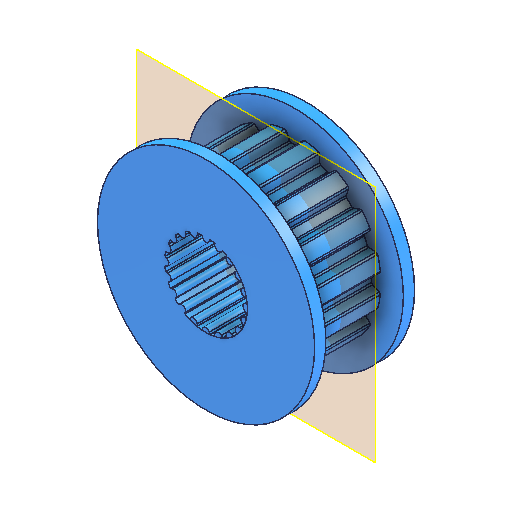
# Autodesk Inventor part: Diff Small Pulley
Saved by Autodesk Inventor 2025.2 (Build 292293000, 293)
## iProperties
Created: 2025-02-20
Part Number: Diff Small Pulley
Material: Generic
Document SubType Name: Modeling
Designer: Jakeg
Density: 1 g/cm^3
Appearance: PTFE
Author: Jakeg
Autodesk Inventor part; units mm, degrees
ref_plane "YZ Plane" through (0, 0, 0) normal (1, 0, 0) x (0, 1, 0)
ref_plane "XZ Plane" through (0, 0, 0) normal (0, 1, 0) x (-1, 0, 0)
ref_plane "XY Plane" through (0, 0, 0) normal (0, 0, 1) x (1, 0, 0)
sketch "Sketch1" plane through (0, 0, 0) normal (0, 0, 1) x (1, 0, 0)
  circle A0 centre (0, 0) radius 6
  circle A1 centre (0, 0) radius 15.75
  dimension "d0" = 12
  dimension "d1" = 31.5
  constraints: 2 centre point, 2 coincident
  measures "d0" diameter of A0
  measures "d1" diameter of A1
extrude "Extrusion1" add sketch "Sketch1" along normal blind 14.5
ref_plane "Work Plane1" through (0, 0, 7.25) normal (0, 0, 1) x (1, 0, 0)
sketch "Sketch2" plane through (0, 0, 7.25) normal (0, 0, 1) x (1, 0, 0)
  circle A0 centre (0, 0) radius 12.5
  circle A1 centre (0, 0) radius 15.75
  dimension "d5" = 25
  constraints: 2 centre point, 2 coincident
  measures "d5" diameter of A0
extrude "Extrusion2" cut sketch "Sketch2" along normal mid plane 11.25
sketch "Sketch3" plane through (0, 0, 14.5) normal (0, 0, 1) x (1, 0, 0)
  arc A0 (-1.278, -5.5468) -> (-2.2269, -5.2385) centre (-1.8276, -5.624) ccw
  arc A1 (-1.2786, -5.8288) -> (-1.278, -5.5468) centre (-2.2683, -5.6858) ccw
  arc A2 (-1.2786, -5.8288) -> (-1.1586, -5.9976) centre (-1.1301, -5.8503) ccw
  arc A3 (-1.1586, -5.9976) -> (-0.7517, -6.062) centre (0, 0) ccw
  arc A4 (-0.7517, -6.062) -> (-0.5855, -5.9386) centre (-0.7333, -5.9131) ccw
  arc A5 (-0.4989, -5.6702) -> (-0.5855, -5.9386) centre (0.4, -6.1084) ccw
  arc A6 (0.4989, -5.6702) -> (-0.4989, -5.6702) centre (0, -5.9134) ccw
  arc A7 (0.5855, -5.9386) -> (0.4989, -5.6702) centre (-0.4, -6.1084) ccw
  arc A8 (0.5855, -5.9386) -> (0.7518, -6.062) centre (0.7333, -5.9131) ccw
  arc A9 (0.7518, -6.062) -> (1.1583, -5.9976) centre (0, 0.0001) ccw
  arc A10 (1.1583, -5.9976) -> (1.2783, -5.8289) centre (1.1299, -5.8503) ccw
  arc A11 (1.2778, -5.5469) -> (1.2783, -5.8289) centre (2.2681, -5.6859) ccw
  arc A12 (2.2267, -5.2385) -> (1.2778, -5.5469) centre (1.8274, -5.624) ccw
  arc A13 (2.392, -5.467) -> (2.2267, -5.2385) centre (1.5072, -5.9331) ccw
  arc A14 (2.392, -5.467) -> (2.5883, -5.533) centre (2.5247, -5.3971) ccw
  arc A15 (2.5883, -5.533) -> (2.955, -5.3461) centre (0, 0.0001) ccw
  arc A16 (2.955, -5.3461) -> (3.017, -5.1486) centre (2.8825, -5.2148) ccw
  arc A17 (2.9293, -4.8805) -> (3.017, -5.1486) centre (3.9141, -4.7067) ccw
  arc A18 (3.7365, -4.2941) -> (2.9293, -4.8805) centre (3.4759, -4.7841) ccw
  arc A19 (3.9643, -4.4603) -> (3.7365, -4.2941) centre (3.2669, -5.1769) ccw
  arc A20 (3.9643, -4.4603) -> (4.1714, -4.4624) centre (4.069, -4.3528) ccw
  arc A21 (4.1714, -4.4624) -> (4.4625, -4.1713) centre (0, 0.0001) ccw
  arc A22 (4.4625, -4.1713) -> (4.4604, -3.9643) centre (4.3529, -4.0689) ccw
  arc A23 (4.2941, -3.7364) -> (4.4604, -3.9643) centre (5.177, -3.2668) ccw
  arc A24 (4.8806, -2.9292) -> (4.2941, -3.7364) centre (4.7841, -3.4758) ccw
  arc A25 (5.1486, -3.0169) -> (4.8806, -2.9292) centre (4.7068, -3.914) ccw
  arc A26 (5.1486, -3.0169) -> (5.3462, -2.9549) centre (5.2149, -2.8824) ccw
  arc A27 (5.3462, -2.9549) -> (5.5331, -2.5882) centre (0, 0.0001) ccw
  arc A28 (5.5331, -2.5882) -> (5.4671, -2.3919) centre (5.3972, -2.5246) ccw
  arc A29 (5.2386, -2.2266) -> (5.4671, -2.3919) centre (5.9331, -1.5071) ccw
  arc A30 (5.5469, -1.2777) -> (5.2386, -2.2266) centre (5.6241, -1.8273) ccw
  arc A31 (5.8289, -1.2783) -> (5.5469, -1.2777) centre (5.6859, -2.268) ccw
  arc A32 (5.8289, -1.2783) -> (5.9977, -1.1582) centre (5.8504, -1.1298) ccw
  arc A33 (5.9977, -1.1582) -> (6.0621, -0.7517) centre (0, 0.0001) ccw
  arc A34 (6.0621, -0.7517) -> (5.9387, -0.5854) centre (5.9132, -0.7332) ccw
  arc A35 (5.6639, -0.4959) -> (5.9387, -0.5854) centre (6.1078, 0.4002) ccw
  arc A36 (5.6639, 0.5019) -> (5.6639, -0.4959) centre (5.9071, 0.003) ccw
  arc A37 (5.9323, 0.5885) -> (5.6639, 0.5019) centre (6.1021, -0.397) ccw
  arc A38 (5.9323, 0.5885) -> (6.0557, 0.7547) centre (5.9068, 0.7363) ccw
  arc A39 (6.0557, 0.7547) -> (5.9913, 1.1613) centre (-0.0064, 0.003) ccw
  arc A40 (5.9913, 1.1613) -> (5.8226, 1.2813) centre (5.844, 1.1329) ccw
  arc A41 (5.5405, 1.2808) -> (5.8226, 1.2813) centre (5.6795, 2.271) ccw
  arc A42 (5.2322, 2.2297) -> (5.5405, 1.2808) centre (5.6177, 1.8304) ccw
  arc A43 (5.4607, 2.395) -> (5.2322, 2.2297) centre (5.9267, 1.5102) ccw
  arc A44 (5.4607, 2.395) -> (5.5267, 2.5912) centre (5.3908, 2.5277) ccw
  arc A45 (5.5267, 2.5912) -> (5.3398, 2.958) centre (-0.0064, 0.003) ccw
  arc A46 (5.3398, 2.958) -> (5.1422, 3.02) centre (5.2085, 2.8854) ccw
  arc A47 (4.8742, 2.9323) -> (5.1422, 3.02) centre (4.7004, 3.9171) ccw
  arc A48 (4.2877, 3.7395) -> (4.8742, 2.9323) centre (4.7777, 3.4789) ccw
  arc A49 (4.454, 3.9673) -> (4.2877, 3.7395) centre (5.1706, 3.2699) ccw
  arc A50 (4.454, 3.9673) -> (4.4561, 4.1744) centre (4.3465, 4.0719) ccw
  arc A51 (4.4561, 4.1744) -> (4.165, 4.4654) centre (-0.0064, 0.003) ccw
  arc A52 (4.165, 4.4654) -> (3.9579, 4.4634) centre (4.0626, 4.3559) ccw
  arc A53 (3.7301, 4.2971) -> (3.9579, 4.4634) centre (3.2605, 5.18) ccw
  arc A54 (2.9229, 4.8836) -> (3.7301, 4.2971) centre (3.4695, 4.7871) ccw
  arc A55 (3.0106, 5.1516) -> (2.9229, 4.8836) centre (3.9077, 4.7098) ccw
  arc A56 (3.0106, 5.1516) -> (2.9486, 5.3492) centre (2.8761, 5.2179) ccw
  arc A57 (2.9486, 5.3492) -> (2.5819, 5.5361) centre (-0.0064, 0.003) ccw
  arc A58 (2.5819, 5.5361) -> (2.3856, 5.4701) centre (2.5183, 5.4002) ccw
  arc A59 (2.2203, 5.2416) -> (2.3856, 5.4701) centre (1.5008, 5.9361) ccw
  arc A60 (1.2714, 5.5499) -> (2.2203, 5.2416) centre (1.821, 5.6271) ccw
  arc A61 (1.2719, 5.8319) -> (1.2714, 5.5499) centre (2.2617, 5.6889) ccw
  arc A62 (1.2719, 5.8319) -> (1.1519, 6.0007) centre (1.1235, 5.8534) ccw
  arc A63 (1.1519, 6.0007) -> (0.7454, 6.0651) centre (-0.0064, 0.003) ccw
  arc A64 (0.7454, 6.0651) -> (0.5791, 5.9417) centre (0.7269, 5.9162) ccw
  arc A65 (0.4925, 5.6733) -> (0.5791, 5.9417) centre (-0.4064, 6.1115) ccw
  arc A66 (-0.5053, 5.6733) -> (0.4925, 5.6733) centre (-0.0064, 5.9165) ccw
  arc A67 (-0.5919, 5.9417) -> (-0.5053, 5.6733) centre (0.3936, 6.1115) ccw
  arc A68 (-0.5919, 5.9417) -> (-0.7581, 6.0651) centre (-0.7397, 5.9162) ccw
  arc A69 (-0.7581, 6.0651) -> (-1.1647, 6.0007) centre (-0.0064, 0.003) ccw
  arc A70 (-1.1647, 6.0007) -> (-1.2847, 5.8319) centre (-1.1363, 5.8534) ccw
  arc A71 (-1.2841, 5.5499) -> (-1.2847, 5.8319) centre (-2.2744, 5.6889) ccw
  arc A72 (-2.2331, 5.2416) -> (-1.2841, 5.5499) centre (-1.8338, 5.6271) ccw
  arc A73 (-2.3984, 5.4701) -> (-2.2331, 5.2416) centre (-1.5136, 5.9361) ccw
  arc A74 (-2.3984, 5.4701) -> (-2.5946, 5.5361) centre (-2.5311, 5.4002) ccw
  arc A75 (-2.5946, 5.5361) -> (-2.9614, 5.3492) centre (-0.0064, 0.003) ccw
  arc A76 (-2.9614, 5.3492) -> (-3.0234, 5.1516) centre (-2.8888, 5.2179) ccw
  arc A77 (-2.9357, 4.8836) -> (-3.0234, 5.1516) centre (-3.9205, 4.7098) ccw
  arc A78 (-3.7429, 4.2971) -> (-2.9357, 4.8836) centre (-3.4823, 4.7871) ccw
  arc A79 (-3.9707, 4.4634) -> (-3.7429, 4.2971) centre (-3.2733, 5.18) ccw
  arc A80 (-3.9707, 4.4634) -> (-4.1778, 4.4654) centre (-4.0753, 4.3559) ccw
  arc A81 (-4.1778, 4.4654) -> (-4.4688, 4.1744) centre (-0.0064, 0.003) ccw
  arc A82 (-4.4688, 4.1744) -> (-4.4667, 3.9673) centre (-4.3592, 4.0719) ccw
  arc A83 (-4.3005, 3.7395) -> (-4.4667, 3.9673) centre (-5.1834, 3.2699) ccw
  arc A84 (-4.887, 2.9323) -> (-4.3005, 3.7395) centre (-4.7905, 3.4789) ccw
  arc A85 (-5.155, 3.02) -> (-4.887, 2.9323) centre (-4.7132, 3.9171) ccw
  arc A86 (-5.155, 3.02) -> (-5.3526, 2.958) centre (-5.2213, 2.8854) ccw
  arc A87 (-5.3526, 2.958) -> (-5.5394, 2.5912) centre (-0.0064, 0.003) ccw
  arc A88 (-5.5394, 2.5912) -> (-5.4735, 2.395) centre (-5.4036, 2.5277) ccw
  arc A89 (-5.245, 2.2297) -> (-5.4735, 2.395) centre (-5.9395, 1.5102) ccw
  arc A90 (-5.5533, 1.2808) -> (-5.245, 2.2297) centre (-5.6305, 1.8304) ccw
  arc A91 (-5.8353, 1.2813) -> (-5.5533, 1.2808) centre (-5.6923, 2.271) ccw
  arc A92 (-5.8353, 1.2813) -> (-6.0041, 1.1613) centre (-5.8568, 1.1329) ccw
  arc A93 (-6.0041, 1.1613) -> (-6.0685, 0.7547) centre (-0.0064, 0.003) ccw
  arc A94 (-6.0685, 0.7547) -> (-5.9451, 0.5885) centre (-5.9196, 0.7363) ccw
  arc A95 (-5.6767, 0.5019) -> (-5.9451, 0.5885) centre (-6.1149, -0.397) ccw
  arc A96 (-5.6767, -0.4959) -> (-5.6767, 0.5019) centre (-5.9199, 0.003) ccw
  arc A97 (-5.9451, -0.5825) -> (-5.6767, -0.4959) centre (-6.1149, 0.403) ccw
  arc A98 (-5.9451, -0.5825) -> (-6.0685, -0.7488) centre (-5.9196, -0.7303) ccw
  arc A99 (-6.0685, -0.7488) -> (-6.0041, -1.1553) centre (-0.0064, 0.003) ccw
  arc A100 (-6.0041, -1.1553) -> (-5.8353, -1.2753) centre (-5.8568, -1.1269) ccw
  arc A101 (-5.5533, -1.2748) -> (-5.8353, -1.2753) centre (-5.6923, -2.2651) ccw
  arc A102 (-5.245, -2.2237) -> (-5.5533, -1.2748) centre (-5.6305, -1.8244) ccw
  arc A103 (-5.4735, -2.389) -> (-5.245, -2.2237) centre (-5.9395, -1.5042) ccw
  arc A104 (-5.4735, -2.389) -> (-5.5394, -2.5853) centre (-5.4036, -2.5217) ccw
  arc A105 (-5.5394, -2.5853) -> (-5.3526, -2.952) centre (-0.0064, 0.003) ccw
  arc A106 (-5.3526, -2.952) -> (-5.155, -3.014) centre (-5.2213, -2.8795) ccw
  arc A107 (-4.887, -2.9263) -> (-5.155, -3.014) centre (-4.7132, -3.9111) ccw
  arc A108 (-4.3005, -3.7335) -> (-4.887, -2.9263) centre (-4.7905, -3.4729) ccw
  arc A109 (-4.4667, -3.9613) -> (-4.3005, -3.7335) centre (-5.1834, -3.2639) ccw
  arc A110 (-4.4667, -3.9613) -> (-4.4688, -4.1684) centre (-4.3592, -4.066) ccw
  arc A111 (-4.4688, -4.1684) -> (-4.1778, -4.4594) centre (-0.0064, 0.003) ccw
  arc A112 (-4.1778, -4.4594) -> (-3.9707, -4.4574) centre (-4.0753, -4.3499) ccw
  arc A113 (-3.7429, -4.2911) -> (-3.9707, -4.4574) centre (-3.2733, -5.174) ccw
  arc A114 (-2.9357, -4.8776) -> (-3.7429, -4.2911) centre (-3.4823, -4.7811) ccw
  arc A115 (-3.0234, -5.1456) -> (-2.9357, -4.8776) centre (-3.9205, -4.7038) ccw
  arc A116 (-3.0234, -5.1456) -> (-2.9614, -5.3432) centre (-2.8888, -5.2119) ccw
  arc A117 (-2.9614, -5.3432) -> (-2.5885, -5.5329) centre (-0.006, 0.0037) ccw
  arc A118 (-2.5885, -5.5329) -> (-2.3922, -5.467) centre (-2.5249, -5.3971) ccw
  arc A119 (-2.2269, -5.2385) -> (-2.3922, -5.467) centre (-1.5074, -5.933) ccw
  circle A120 centre (-0.006, 0.0037) radius 6
  circle A121 centre (-0.006, 0.0037) radius 12.5204
  arc A122 (-9.7164, 7.9073) -> (-9.7028, 7.7034) centre (-9.6001, 7.8127) ccw
  arc A123 (-9.5366, 7.4755) -> (-9.7028, 7.7034) centre (-10.4195, 7.0059) ccw
  arc A124 (-10.1231, 6.6683) -> (-9.5366, 7.4755) centre (-10.0266, 7.2149) ccw
  arc A125 (-10.3911, 6.756) -> (-10.1231, 6.6683) centre (-9.9492, 7.6531) ccw
  arc A126 (-10.3911, 6.756) -> (-10.5841, 6.7017) centre (-10.4574, 6.6215) ccw
  arc A127 (-11.383, 4.9039) -> (-11.5641, 4.8177) centre (-11.4256, 4.76) ccw
  arc A128 (-11.383, 4.9039) -> (-11.104, 4.8627) centre (-11.0991, 5.8627) ccw
  arc A129 (-11.104, 4.8627) -> (-10.6624, 5.7574) centre (-11.1013, 5.4177) ccw
  arc A130 (-10.9126, 6.1526) -> (-10.8647, 5.9539) centre (-10.7819, 6.079) ccw
  arc A131 (-10.6624, 5.7574) -> (-10.8647, 5.9539) centre (-11.4532, 5.1454) ccw
  arc A132 (-12.0476, 2.9107) -> (-12.2115, 2.7952) centre (-12.0653, 2.7618) ccw
  arc A133 (-12.0476, 2.9107) -> (-11.7657, 2.9173) centre (-11.9298, 3.9038) ccw
  arc A134 (-11.7657, 2.9173) -> (-11.4816, 3.8738) centre (-11.8568, 3.4648) ccw
  arc A135 (-11.795, 4.221) -> (-11.7143, 4.0332) centre (-11.6538, 4.1705) ccw
  arc A136 (-11.4816, 3.8738) -> (-11.7143, 4.0332) centre (-12.1576, 3.1369) ccw
  arc A137 (-12.3658, 0.8339) -> (-12.5078, 0.6924) centre (-12.3581, 0.6841) ccw
  arc A138 (-12.3658, 0.8339) -> (-12.0891, 0.8881) centre (-12.4176, 1.8326) ccw
  arc A139 (-12.0891, 0.8881) -> (-11.9707, 1.8788) centre (-12.2714, 1.4123) ccw
  arc A140 (-12.3383, 2.1681) -> (-12.227, 1.9966) centre (-12.1906, 2.1421) ccw
  arc A141 (-11.9707, 1.8788) -> (-12.227, 1.9966) centre (-12.5124, 1.0382) ccw
  arc A142 (-12.3285, -1.2668) -> (-12.4445, -1.4303) centre (-12.2955, -1.4131) ccw
  arc A143 (-12.3285, -1.2668) -> (-12.0648, -1.1666) centre (-12.5483, -0.2912) ccw
  arc A144 (-12.0648, -1.1666) -> (-12.1157, -0.1702) centre (-12.3331, -0.6808) ccw
  arc A145 (-12.5268, 0.0528) -> (-12.3881, -0.0974) centre (-12.3768, 0.0522) ccw
  arc A146 (-12.1157, -0.1702) -> (-12.3881, -0.0974) centre (-12.5075, -1.0902) ccw
  arc A147 (-11.9366, -3.331) -> (-12.0234, -3.5117) centre (-11.8794, -3.4696) ccw
  arc A148 (-11.9366, -3.331) -> (-11.6937, -3.1877) centre (-12.3181, -2.4066) ccw
  arc A149 (-11.6937, -3.1877) -> (-11.9122, -2.2142) centre (-12.0403, -2.7542) ccw
  arc A150 (-12.3551, -2.0639) -> (-12.193, -2.1884) centre (-12.2072, -2.0391) ccw
  arc A151 (-11.9122, -2.2142) -> (-12.193, -2.1884) centre (-12.1429, -3.1872) ccw
  arc A152 (-11.2016, -5.2992) -> (-11.2565, -5.4921) centre (-11.1218, -5.4262) ccw
  arc A153 (-11.2016, -5.2992) -> (-10.9864, -5.117) centre (-11.7338, -4.4526) ccw
  arc A154 (-10.9864, -5.117) -> (-11.3663, -4.1944) centre (-11.4012, -4.7483) ccw
  arc A155 (-11.8282, -4.1211) -> (-11.6474, -4.2165) centre (-11.6866, -4.0717) ccw
  arc A156 (-11.3663, -4.1944) -> (-11.6474, -4.2165) centre (-11.4292, -5.1924) ccw
  arc A157 (-10.1445, -7.115) -> (-10.166, -7.3143) centre (-10.0443, -7.2266) ccw
  arc A158 (-10.1445, -7.115) -> (-9.9632, -6.899) centre (-10.8121, -6.3705) ccw
  arc A159 (-9.9632, -6.899) -> (-10.4935, -6.0538) centre (-10.4343, -6.6057) ccw
  arc A160 (-10.9612, -6.0597) -> (-10.7669, -6.1231) centre (-10.83, -5.987) ccw
  arc A161 (-10.4935, -6.0538) -> (-10.7669, -6.1231) centre (-10.3869, -7.0481) ccw
  arc A162 (-8.7957, -8.7259) -> (-8.7833, -8.926) centre (-8.6781, -8.8191) ccw
  arc A163 (-8.7957, -8.7259) -> (-8.6535, -8.4824) centre (-9.5796, -8.105) ccw
  arc A164 (-8.6535, -8.4824) -> (-9.319, -7.739) centre (-9.1675, -8.2729) ccw
  arc A165 (-9.779, -7.8238) -> (-9.5768, -7.8535) centre (-9.662, -7.7301) ccw
  arc A166 (-9.319, -7.739) -> (-9.5768, -7.8535) centre (-9.0459, -8.701) ccw
  arc A167 (-7.1941, -10.0858) -> (-7.148, -10.2809) centre (-7.0625, -10.1577) ccw
  arc A168 (-7.1941, -10.0858) -> (-7.0951, -9.8217) centre (-8.0716, -9.6062) ccw
  arc A169 (-7.0951, -9.8217) -> (-7.8767, -9.2015) centre (-7.6371, -9.7021) ccw
  arc A170 (-8.3157, -9.3628) -> (-8.1113, -9.3579) centre (-8.2162, -9.2506) ccw
  arc A171 (-7.8767, -9.2015) -> (-8.1113, -9.3579) centre (-7.4449, -10.1035) ccw
  arc A172 (-5.3857, -11.1554) -> (-5.3073, -11.3399) centre (-5.2438, -11.204) ccw
  arc A173 (-5.3857, -11.1554) -> (-5.3328, -10.8784) centre (-6.3316, -10.831) ccw
  arc A174 (-5.3328, -10.8784) -> (-6.2079, -10.3992) centre (-5.8871, -10.8521) ccw
  arc A175 (-6.6134, -10.6324) -> (-6.4128, -10.593) centre (-6.5342, -10.505) ccw
  arc A176 (-6.2079, -10.3992) -> (-6.4128, -10.593) centre (-5.6299, -11.2153) ccw
  arc A177 (-3.4225, -11.904) -> (-3.3141, -12.0726) centre (-3.2745, -11.9279) ccw
  arc A178 (-3.4225, -11.904) -> (-3.4172, -11.622) centre (-4.4097, -11.7442) ccw
  arc A179 (-3.4172, -11.622) -> (-4.3607, -11.2976) centre (-3.968, -11.6898) ccw
  arc A180 (-4.7209, -11.596) -> (-4.5299, -11.5233) centre (-4.6645, -11.457) ccw
  arc A181 (-4.3607, -11.2976) -> (-4.5299, -11.5233) centre (-3.6531, -12.0043) ccw
  arc A182 (-1.3611, -12.31) -> (-1.2257, -12.4579) centre (-1.2111, -12.3086) ccw
  arc A183 (-1.3611, -12.31) -> (-1.4035, -12.0312) centre (-2.3611, -12.3194) ccw
  arc A184 (-1.4035, -12.0312) -> (-2.3883, -11.871) centre (-1.9349, -12.1911) ccw
  arc A185 (-2.6929, -12.2259) -> (-2.5169, -12.122) centre (-2.6607, -12.0794) ccw
  arc A186 (-2.3883, -11.871) -> (-2.5169, -12.122) centre (-1.5715, -12.4479) ccw
  arc A187 (0.7393, -12.3619) -> (0.8977, -12.4848) centre (0.8869, -12.3352) ccw
  arc A188 (0.7393, -12.3619) -> (0.6504, -12.0942) centre (-0.2447, -12.5401) ccw
  arc A189 (0.6504, -12.0942) -> (-0.3473, -12.1027) centre (0.1536, -12.3417) ccw
  arc A190 (-0.5875, -12.5041) -> (-0.4316, -12.3718) centre (-0.5806, -12.3542) ccw
  arc A191 (-0.3473, -12.1027) -> (-0.4316, -12.3718) centre (0.5553, -12.5333) ccw
  arc A192 (2.8182, -12.058) -> (2.9952, -12.1523) centre (2.9592, -12.0067) ccw
  arc A193 (2.8182, -12.058) -> (2.6854, -11.8092) centre (1.8785, -12.3999) ccw
  arc A194 (2.6854, -11.8092) -> (1.7035, -11.9862) centre (2.2376, -12.1371) ccw
  arc A195 (1.5345, -12.4224) -> (1.6658, -12.2657) centre (1.5161, -12.2735) ccw
  arc A196 (1.7035, -11.9862) -> (1.6658, -12.2657) centre (2.6658, -12.258) ccw
  arc A197 (4.8159, -11.4072) -> (5.0062, -11.4702) centre (4.9462, -11.3328) ccw
  arc A198 (4.8159, -11.4072) -> (4.643, -11.1844) centre (3.9475, -11.903) ccw
  arc A199 (4.643, -11.1844) -> (3.7051, -11.5248) centre (4.257, -11.5832) ccw
  arc A200 (3.6123, -11.9832) -> (3.7152, -11.8066) centre (3.5689, -11.8396) ccw
  arc A201 (3.7051, -11.5248) -> (3.7152, -11.8066) centre (4.6995, -11.6301) ccw
  arc A202 (6.6749, -10.4281) -> (6.8731, -10.4581) centre (6.7907, -10.3327) ccw
  arc A203 (6.6749, -10.4281) -> (6.4668, -10.2377) centre (5.9027, -11.0635) ccw
  arc A204 (6.4668, -10.2377) -> (5.5999, -10.7317) centre (6.1537, -10.696) ccw
  arc A205 (5.5859, -11.1993) -> (5.6575, -11.0078) centre (5.5189, -11.0651) ccw
  arc A206 (5.5999, -10.7317) -> (5.6575, -11.0078) centre (6.5978, -10.6674) ccw
  arc A207 (8.3416, -9.1489) -> (8.5421, -9.1449) centre (8.4397, -9.0354) ccw
  arc A208 (8.3416, -9.1489) -> (8.1044, -8.9965) centre (7.688, -9.9057) ccw
  arc A209 (8.1044, -8.9965) -> (7.3334, -9.6299) centre (7.8733, -9.5011) ccw
  arc A210 (7.3986, -10.093) -> (7.4369, -9.8922) centre (7.3099, -9.9721) ccw
  arc A211 (7.3334, -9.6299) -> (7.4369, -9.8922) centre (8.3061, -9.3978) ccw
  arc A212 (9.7682, -7.6064) -> (9.9651, -7.5687) centre (9.8457, -7.478) ccw
  arc A213 (9.7682, -7.6064) -> (9.5086, -7.4963) centre (9.2519, -8.4628) ccw
  arc A214 (9.5086, -7.4963) -> (8.8558, -8.2509) centre (9.3661, -8.0327) ccw
  arc A215 (8.9984, -8.6963) -> (9.0021, -8.4919) centre (8.8905, -8.5921) ccw
  arc A216 (8.8558, -8.2509) -> (9.0021, -8.4919) centre (9.7753, -7.8578) ccw
  arc A217 (10.9136, -5.845) -> (11.1013, -5.7745) centre (10.9683, -5.7053) ccw
  arc A218 (10.9136, -5.845) -> (10.6391, -5.7804) centre (10.5494, -6.7764) ccw
  arc A219 (10.6391, -5.7804) -> (10.1232, -6.6344) centre (10.5893, -6.3332) ccw
  arc A220 (10.339, -7.0494) -> (10.3082, -6.8473) centre (10.2151, -6.9649) ccw
  arc A221 (10.1232, -6.6344) -> (10.3082, -6.8473) centre (10.9631, -6.0916) ccw
  arc A222 (11.7449, -3.9154) -> (11.918, -3.8142) centre (11.7751, -3.7685) ccw
  arc A223 (11.7449, -3.9154) -> (11.4634, -3.8981) centre (11.5433, -4.8949) ccw
  arc A224 (11.4634, -3.8981) -> (11.0993, -4.827) centre (11.5078, -4.4513) ccw
  arc A225 (11.3821, -5.1996) -> (11.3175, -5.0056) centre (11.2456, -5.1373) ccw
  arc A226 (11.0993, -4.827) -> (11.3175, -5.0056) centre (11.8353, -4.1501) ccw
  arc A227 (12.2381, -1.8731) -> (12.3916, -1.7441) centre (12.243, -1.7232) ccw
  arc A228 (12.2381, -1.8731) -> (11.9577, -1.9036) centre (12.2049, -2.8725) ccw
  arc A229 (11.9577, -1.9036) -> (11.7558, -2.8807) centre (12.0949, -2.4414) ccw
  arc A230 (12.0975, -3.2001) -> (12.0011, -3.0198) centre (11.9525, -3.1617) ccw
  arc A231 (11.7558, -2.8807) -> (12.0011, -3.0198) centre (12.3668, -2.0891) ccw
  arc A232 (12.379, 0.2232) -> (12.5085, 0.3763) centre (12.3586, 0.3718) ccw
  arc A233 (12.379, 0.2232) -> (12.1078, 0.1458) centre (12.5153, -0.7675) ccw
  arc A234 (12.1078, 0.1458) -> (12.0739, -0.8514) centre (12.3339, -0.3611) ccw
  arc A235 (12.4647, -1.1084) -> (12.3392, -0.9471) centre (12.3153, -1.0951) ccw
  arc A236 (12.0739, -0.8514) -> (12.3392, -0.9471) centre (12.5424, 0.0321) ccw
  arc A237 (12.1636, 2.3132) -> (12.2654, 2.486) centre (12.1184, 2.4562) ccw
  arc A238 (12.1636, 2.3132) -> (11.9094, 2.191) centre (12.4653, 1.3598) ccw
  arc A239 (11.9094, 2.191) -> (12.0446, 1.2025) centre (12.218, 1.7297) ccw
  arc A240 (12.4732, 1.0152) -> (12.3222, 1.153) centre (12.3237, 1.003) ccw
  arc A241 (12.0446, 1.2025) -> (12.3222, 1.153) centre (12.357, 2.1524) ccw
  arc A242 (11.5981, 4.3367) -> (11.6692, 4.5242) centre (11.5294, 4.47) ccw
  arc A243 (11.5981, 4.3367) -> (11.3683, 4.1733) centre (12.0567, 3.448) ccw
  arc A244 (11.3683, 4.1733) -> (11.6685, 3.2218) centre (11.7503, 3.7708) ccw
  arc A245 (12.1226, 3.1097) -> (11.9505, 3.22) centre (11.9773, 3.0724) ccw
  arc A246 (11.6685, 3.2218) -> (11.9505, 3.22) centre (11.8159, 4.2109) ccw
  arc A247 (10.6988, 6.2355) -> (10.7372, 6.4323) centre (10.6085, 6.3553) ccw
  arc A248 (10.6988, 6.2355) -> (10.4999, 6.0357) centre (11.3009, 5.4371) ccw
  arc A249 (10.4999, 6.0357) -> (10.9566, 5.1486) centre (10.9444, 5.7035) ccw
  arc A250 (11.4231, 5.1148) -> (11.2348, 5.1945) centre (11.2862, 5.0535) ccw
  arc A251 (10.9566, 5.1486) -> (11.2348, 5.1945) centre (10.9347, 6.1484) ccw
  arc A252 (9.4915, 7.9551) -> (9.4961, 8.1555) centre (9.3823, 8.0579) ccw
  arc A253 (9.4915, 7.9551) -> (9.3292, 7.7245) centre (10.2199, 7.2699) ccw
  arc A254 (9.3292, 7.7245) -> (9.9293, 6.9274) centre (9.8235, 7.4722) ccw
  arc A255 (10.3948, 6.9729) -> (10.1958, 7.0196) centre (10.2702, 6.8893) ccw
  arc A256 (9.9293, 6.9274) -> (10.1958, 7.0196) centre (9.7388, 7.909) ccw
  arc A257 (8.011, 9.4458) -> (7.9816, 9.6442) centre (7.886, 9.5287) ccw
  arc A258 (8.011, 9.4458) -> (7.89, 9.1911) centre (8.8447, 8.8936) ccw
  arc A259 (7.89, 9.1911) -> (8.6162, 8.5069) centre (8.4199, 9.026) ccw
  arc A260 (9.0673, 8.6304) -> (8.8632, 8.6428) centre (8.9586, 8.527) ccw
  arc A261 (8.6162, 8.5069) -> (8.8632, 8.6428) centre (8.2625, 9.4422) ccw
  arc A262 (6.2998, 10.665) -> (6.2374, 10.8555) centre (6.1626, 10.7255) ccw
  arc A263 (6.2998, 10.665) -> (6.2236, 10.3935) centre (7.2149, 10.2616) ccw
  arc A264 (6.2236, 10.3935) -> (7.055, 9.8418) centre (6.7737, 10.3203) ccw
  arc A265 (7.4787, 10.0398) -> (7.2755, 10.0175) centre (7.3891, 9.9195) ccw
  arc A266 (7.055, 9.8418) -> (7.2755, 10.0175) centre (6.5483, 10.7039) ccw
  arc A267 (4.4072, 11.5774) -> (4.3135, 11.7546) centre (4.2617, 11.6138) ccw
  arc A268 (4.4072, 11.5774) -> (4.378, 11.2969) centre (5.3773, 11.3344) ccw
  arc A269 (4.378, 11.2969) -> (5.2906, 10.8936) centre (4.9326, 11.3177) ccw
  arc A270 (5.6748, 11.1604) -> (5.4783, 11.1041) centre (5.6068, 11.0267) ccw
  arc A271 (5.2906, 10.8936) -> (5.4783, 11.1041) centre (4.6455, 11.6577) ccw
  arc A272 (2.3877, 12.1568) -> (2.2653, 12.3156) centre (2.2381, 12.1681) ccw
  arc A273 (2.3877, 12.1568) -> (2.4062, 11.8754) centre (3.3848, 12.0813) ccw
  arc A274 (2.4062, 11.8754) -> (3.3739, 11.6322) centre (2.9494, 11.9896) ccw
  arc A275 (3.7075, 11.96) -> (3.5233, 11.8714) centre (3.663, 11.8168) ccw
  arc A276 (3.3739, 11.6322) -> (3.5233, 11.8714) centre (2.609, 12.2763) ccw
  arc A277 (0.2992, 12.3866) -> (0.1518, 12.5224) centre (0.1499, 12.3724) ccw
  arc A278 (0.2992, 12.3866) -> (0.3651, 12.1123) centre (1.2948, 12.4806) ccw
  arc A279 (0.3651, 12.1123) -> (1.3599, 12.0362) centre (0.8811, 12.3168) ccw
  arc A280 (1.6333, 12.4157) -> (1.4668, 12.2972) centre (1.6137, 12.267) ccw
  arc A281 (1.3599, 12.0362) -> (1.4668, 12.2972) centre (0.4971, 12.5417) ccw
  arc A282 (-1.798, 12.2601) -> (-1.9663, 12.3691) centre (-1.9428, 12.2209) ccw
  arc A283 (-1.798, 12.2601) -> (-1.6867, 12.0009) centre (-0.8326, 12.5211) ccw
  arc A284 (-1.6867, 12.0009) -> (-0.6933, 12.094) centre (-1.2127, 12.2896) ccw
  arc A285 (-0.488, 12.5143) -> (-0.6321, 12.3693) centre (-0.4822, 12.3644) ccw
  arc A286 (-0.6933, 12.094) -> (-0.6321, 12.3693) centre (-1.6292, 12.4465) ccw
  arc A287 (-3.8437, 11.781) -> (-4.028, 11.86) centre (-3.9798, 11.7179) ccw
  arc A288 (-3.8437, 11.781) -> (-3.6902, 11.5444) centre (-2.9363, 12.2014) ccw
  arc A289 (-3.6902, 11.5444) -> (-2.7268, 11.804) centre (-3.2718, 11.909) ccw
  arc A290 (-2.5955, 12.2529) -> (-2.7131, 12.0857) centre (-2.5645, 12.1062) ccw
  arc A291 (-2.7268, 11.804) -> (-2.7131, 12.0857) centre (-3.7088, 11.9932) ccw
  arc A292 (-5.779, 10.9631) -> (-5.974, 11.0098) centre (-5.9025, 10.8779) ccw
  arc A293 (-5.779, 10.9631) -> (-5.5877, 10.7558) centre (-4.9557, 11.5307) ccw
  arc A294 (-5.5877, 10.7558) -> (-4.6821, 11.1745) centre (-5.237, 11.1859) ccw
  arc A295 (-4.6285, 11.6391) -> (-4.7161, 11.4544) centre (-4.5731, 11.4997) ccw
  arc A296 (-4.6821, 11.1745) -> (-4.7161, 11.4544) centre (-5.6819, 11.195) ccw
  arc A297 (-7.5482, 9.8299) -> (-7.7483, 9.8429) centre (-7.6555, 9.7251) ccw
  arc A298 (-7.5482, 9.8299) -> (-7.3247, 9.6579) centre (-6.8327, 10.5285) ccw
  arc A299 (-7.3247, 9.6579) -> (-6.5028, 10.2236) centre (-7.0517, 10.1411) ccw
  arc A300 (-6.5285, 10.6906) -> (-6.5837, 10.4938) centre (-6.4504, 10.5626) ccw
  arc A301 (-6.5028, 10.2236) -> (-6.5837, 10.4938) centre (-7.4917, 10.0749) ccw
  arc A302 (-9.1005, 8.4139) -> (-9.2999, 8.393) centre (-9.1885, 8.2925) ccw
  arc A303 (-9.1005, 8.4139) -> (-8.8511, 8.2822) centre (-8.5134, 9.2234) ccw
  arc A304 (-8.8511, 8.2822) -> (-8.1367, 8.9787) centre (-8.6637, 8.8046) ccw
  arc A305 (-8.2409, 9.4347) -> (-8.262, 9.2313) centre (-8.1423, 9.3217) ccw
  arc A306 (-8.1367, 8.9787) -> (-8.262, 9.2313) centre (-9.0862, 8.665) ccw
  point P0 (-3.9961, -4.4772)
  point P1 (-3.0344, -5.1759)
  point P2 (-5.1854, -3.0251)
  point P3 (-4.4866, -3.9867)
  point P4 (-5.8678, -1.2765)
  point P5 (-5.5003, -2.4071)
  point P6 (-5.9765, 0.5975)
  point P7 (-5.9764, -0.5915)
  point P8 (-5.5008, 2.4135)
  point P9 (-5.8681, 1.2824)
  point P10 (-4.4872, 3.9936)
  point P11 (-5.1861, 3.0313)
  point P12 (-3.0348, 5.1832)
  point P13 (-3.9971, 4.4838)
  point P14 (-1.2858, 5.8657)
  point P15 (-2.4173, 5.4979)
  point P16 (0.5886, 5.9742)
  point P17 (-0.6013, 5.9741)
  point P18 (2.4047, 5.4982)
  point P19 (1.273, 5.8659)
  point P20 (3.9848, 4.4841)
  point P21 (3.0221, 5.1836)
  point P22 (5.1741, 3.0314)
  point P23 (4.4747, 3.9941)
  point P24 (5.8562, 1.2824)
  point P25 (5.4886, 2.414)
  point P26 (5.9644, -0.5922)
  point P27 (5.9645, 0.5978)
  point P28 (5.4889, -2.4059)
  point P29 (5.8551, -1.2797)
  point P30 (4.4768, -3.9843)
  point P31 (5.1727, -3.0263)
  point P32 (3.0266, -5.1734)
  point P33 (3.9846, -4.4768)
  point P34 (1.2797, -5.8569)
  point P35 (2.4067, -5.4898)
  point P36 (-0.5935, -5.9674)
  point P37 (0.593, -5.9663)
  point P38 (-2.4101, -5.4936)
  point P39 (-1.2798, -5.8595)
  dimension "d8" = 0
  dimension "d9" = 0
  dimension "d20" = 360
  constraints: 612 point on circle, 306 centre point, 3 coincident, 2 tangent, 595 other
  measures "d8" distance of point (0, 0) point (0, 0)
  measures "d9" distance of point (0, 0) point (0, 0)
extrude "Extrusion3" add sketch "Sketch3" against normal blind 14.5 contours A1 A2 A120 A118 A119 A0 | A120 A4 A3 A2 | A118 A117 A116 A120 | A4 A5 A6 A7 A8 A120 | A120 A112 A113 A114 A115 A116 | A120 A10 A9 A8 | A112 A111 A110 A120 | A10 A11 A12 A13 A14 A120 | A120 A106 A107 A108 A109 A110 | A120 A16 A15 A14 | A106 A105 A104 A120 | A16 A17 A18 A19 A20 A120 | A120 A100 A101 A102 A103 A104 | A120 A22 A21 A20 | A100 A99 A98 A120 | A22 A23 A24 A25 A26 A120 | A120 A94 A95 A96 A97 A98 | A120 A28 A27 A26 | A94 A93 A92 A120 | A28 A29 A30 A31 A32 A120 | A120 A88 A89 A90 A91 A92 | A120 A34 A33 A32 | A88 A87 A86 A120 | A34 A35 A36 A37 A38 A120 | A120 A82 A83 A84 A85 A86 | A82 A81 A80 A120 | A120 A40 A39 A38 | A120 A76 A77 A78 A79 A80 | A40 A41 A42 A43 A44 A120 | A76 A75 A74 A120 | A120 A46 A45 A44 | A120 A70 A71 A72 A73 A74 | A46 A47 A48 A49 A50 A120 | A70 A69 A68 A120 | A120 A52 A51 A50 | A120 A64 A65 A66 A67 A68 | A52 A53 A54 A55 A56 A120 | A64 A63 A62 A120 | A120 A58 A57 A56 | A120 A58 A59 A60 A61 A62
sketch "Sketch6" plane through (0, 0, 1.625) normal (0, 0, 1) x (1, 0, 0)
  circle A0 centre (0, 0) radius 14.7498
  line L0 (3.5809, 11.7957) -> (3.627, 10.7394)
  arc A1 (3.627, 10.7394) -> (3.7836, 10.5159) centre (3.8808, 10.7505) ccw
  line L1 (3.7836, 10.5159) -> (4.7604, 10.1112)
  arc A2 (4.7604, 10.1112) -> (5.0292, 10.1586) centre (4.8576, 10.3459) ccw
  line L2 (5.0292, 10.1586) -> (5.8087, 10.8729)
  arc A3 (6.1044, 10.9073) -> (5.8087, 10.8729) centre (5.9803, 10.6856) ccw
  arc A4 (7.741, 9.8138) -> (6.1044, 10.9073) centre (0, 0) ccw
  arc A5 (7.8223, 9.5275) -> (7.741, 9.8138) centre (7.5837, 9.6143) ccw
  line L3 (7.8223, 9.5275) -> (7.4607, 8.534)
  arc A6 (7.4607, 8.534) -> (7.5198, 8.2675) centre (7.6994, 8.4471) ccw
  line L4 (7.5198, 8.2675) -> (8.2675, 7.5198)
  arc A7 (8.2675, 7.5198) -> (8.534, 7.4607) centre (8.4471, 7.6994) ccw
  line L5 (8.534, 7.4607) -> (9.5275, 7.8223)
  arc A8 (9.8138, 7.741) -> (9.5275, 7.8223) centre (9.6143, 7.5837) ccw
  arc A9 (10.9073, 6.1044) -> (9.8138, 7.741) centre (0, 0) ccw
  arc A10 (10.8729, 5.8087) -> (10.9073, 6.1044) centre (10.6856, 5.9803) ccw
  line L6 (10.8729, 5.8087) -> (10.1586, 5.0292)
  arc A11 (10.1586, 5.0292) -> (10.1112, 4.7604) centre (10.3459, 4.8576) ccw
  line L7 (10.1112, 4.7604) -> (10.5159, 3.7836)
  arc A12 (10.5159, 3.7836) -> (10.7394, 3.627) centre (10.7505, 3.8808) ccw
  line L8 (10.7394, 3.627) -> (11.7957, 3.5809)
  arc A13 (12.0291, 3.3962) -> (11.7957, 3.5809) centre (11.7846, 3.3271) ccw
  arc A14 (12.4131, 1.4657) -> (12.0291, 3.3962) centre (0, 0) ccw
  arc A15 (12.2682, 1.2057) -> (12.4131, 1.4657) centre (12.1608, 1.4359) ccw
  line L9 (12.2682, 1.2057) -> (11.31, 0.7589)
  arc A16 (11.31, 0.7589) -> (11.1633, 0.5287) centre (11.4173, 0.5287) ccw
  line L10 (11.1633, 0.5287) -> (11.1633, -0.5287)
  arc A17 (11.1633, -0.5287) -> (11.31, -0.7589) centre (11.4173, -0.5287) ccw
  line L11 (11.31, -0.7589) -> (12.2682, -1.2057)
  arc A18 (12.4131, -1.4657) -> (12.2682, -1.2057) centre (12.1608, -1.4359) ccw
  arc A19 (12.0291, -3.3962) -> (12.4131, -1.4657) centre (0, 0) ccw
  arc A20 (11.7957, -3.5809) -> (12.0291, -3.3962) centre (11.7846, -3.3271) ccw
  line L12 (11.7957, -3.5809) -> (10.7394, -3.627)
  arc A21 (10.7394, -3.627) -> (10.5159, -3.7836) centre (10.7505, -3.8808) ccw
  line L13 (10.5159, -3.7836) -> (10.1112, -4.7604)
  arc A22 (10.1112, -4.7604) -> (10.1586, -5.0292) centre (10.3459, -4.8576) ccw
  line L14 (10.1586, -5.0292) -> (10.8729, -5.8087)
  arc A23 (10.9073, -6.1044) -> (10.8729, -5.8087) centre (10.6856, -5.9803) ccw
  arc A24 (9.8138, -7.741) -> (10.9073, -6.1044) centre (0, 0) ccw
  arc A25 (9.5275, -7.8223) -> (9.8138, -7.741) centre (9.6143, -7.5837) ccw
  line L15 (9.5275, -7.8223) -> (8.534, -7.4607)
  arc A26 (8.534, -7.4607) -> (8.2675, -7.5198) centre (8.4471, -7.6994) ccw
  line L16 (8.2675, -7.5198) -> (7.5198, -8.2675)
  arc A27 (7.5198, -8.2675) -> (7.4607, -8.534) centre (7.6994, -8.4471) ccw
  line L17 (7.4607, -8.534) -> (7.8223, -9.5275)
  arc A28 (7.741, -9.8138) -> (7.8223, -9.5275) centre (7.5837, -9.6143) ccw
  arc A29 (6.1044, -10.9073) -> (7.741, -9.8138) centre (0, 0) ccw
  arc A30 (5.8087, -10.8729) -> (6.1044, -10.9073) centre (5.9803, -10.6856) ccw
  line L18 (5.8087, -10.8729) -> (5.0292, -10.1586)
  arc A31 (5.0292, -10.1586) -> (4.7604, -10.1112) centre (4.8576, -10.3459) ccw
  line L19 (4.7604, -10.1112) -> (3.7836, -10.5159)
  arc A32 (3.7836, -10.5159) -> (3.627, -10.7394) centre (3.8808, -10.7505) ccw
  line L20 (3.627, -10.7394) -> (3.5809, -11.7957)
  arc A33 (3.3962, -12.0291) -> (3.5809, -11.7957) centre (3.3271, -11.7846) ccw
  arc A34 (1.4657, -12.4131) -> (3.3962, -12.0291) centre (0, 0) ccw
  arc A35 (1.2057, -12.2682) -> (1.4657, -12.4131) centre (1.4359, -12.1608) ccw
  line L21 (1.2057, -12.2682) -> (0.7589, -11.31)
  arc A36 (0.7589, -11.31) -> (0.5287, -11.1633) centre (0.5287, -11.4173) ccw
  line L22 (0.5287, -11.1633) -> (-0.5287, -11.1633)
  arc A37 (-0.5287, -11.1633) -> (-0.7589, -11.31) centre (-0.5287, -11.4173) ccw
  line L23 (-0.7589, -11.31) -> (-1.2057, -12.2682)
  arc A38 (-1.4657, -12.4131) -> (-1.2057, -12.2682) centre (-1.4359, -12.1608) ccw
  arc A39 (-3.3962, -12.0291) -> (-1.4657, -12.4131) centre (0, 0) ccw
  arc A40 (-3.5809, -11.7957) -> (-3.3962, -12.0291) centre (-3.3271, -11.7846) ccw
  line L24 (-3.5809, -11.7957) -> (-3.627, -10.7394)
  arc A41 (-3.627, -10.7394) -> (-3.7836, -10.5159) centre (-3.8808, -10.7505) ccw
  line L25 (-3.7836, -10.5159) -> (-4.7604, -10.1112)
  arc A42 (-4.7604, -10.1112) -> (-5.0292, -10.1586) centre (-4.8576, -10.3459) ccw
  line L26 (-5.0292, -10.1586) -> (-5.8087, -10.8729)
  arc A43 (-6.1044, -10.9073) -> (-5.8087, -10.8729) centre (-5.9803, -10.6856) ccw
  arc A44 (-7.741, -9.8138) -> (-6.1044, -10.9073) centre (0, 0) ccw
  arc A45 (-7.8223, -9.5275) -> (-7.741, -9.8138) centre (-7.5837, -9.6143) ccw
  line L27 (-7.8223, -9.5275) -> (-7.4607, -8.534)
  arc A46 (-7.4607, -8.534) -> (-7.5198, -8.2675) centre (-7.6994, -8.4471) ccw
  line L28 (-7.5198, -8.2675) -> (-8.2675, -7.5198)
  arc A47 (-8.2675, -7.5198) -> (-8.534, -7.4607) centre (-8.4471, -7.6994) ccw
  line L29 (-8.534, -7.4607) -> (-9.5275, -7.8223)
  arc A48 (-9.8138, -7.741) -> (-9.5275, -7.8223) centre (-9.6143, -7.5837) ccw
  arc A49 (-10.9073, -6.1044) -> (-9.8138, -7.741) centre (0, 0) ccw
  arc A50 (-10.8729, -5.8087) -> (-10.9073, -6.1044) centre (-10.6856, -5.9803) ccw
  line L30 (-10.8729, -5.8087) -> (-10.1586, -5.0292)
  arc A51 (-10.1586, -5.0292) -> (-10.1112, -4.7604) centre (-10.3459, -4.8576) ccw
  line L31 (-10.1112, -4.7604) -> (-10.5159, -3.7836)
  arc A52 (-10.5159, -3.7836) -> (-10.7394, -3.627) centre (-10.7505, -3.8808) ccw
  line L32 (-10.7394, -3.627) -> (-11.7957, -3.5809)
  arc A53 (-12.0291, -3.3962) -> (-11.7957, -3.5809) centre (-11.7846, -3.3271) ccw
  arc A54 (-12.4131, -1.4657) -> (-12.0291, -3.3962) centre (0, 0) ccw
  arc A55 (-12.2682, -1.2057) -> (-12.4131, -1.4657) centre (-12.1608, -1.4359) ccw
  line L33 (-12.2682, -1.2057) -> (-11.31, -0.7589)
  arc A56 (-11.31, -0.7589) -> (-11.1633, -0.5287) centre (-11.4173, -0.5287) ccw
  line L34 (-11.1633, -0.5287) -> (-11.1633, 0.5287)
  arc A57 (-11.1633, 0.5287) -> (-11.31, 0.7589) centre (-11.4173, 0.5287) ccw
  line L35 (-11.31, 0.7589) -> (-12.2682, 1.2057)
  arc A58 (-12.4131, 1.4657) -> (-12.2682, 1.2057) centre (-12.1608, 1.4359) ccw
  arc A59 (-12.0291, 3.3962) -> (-12.4131, 1.4657) centre (0, 0) ccw
  arc A60 (-11.7957, 3.5809) -> (-12.0291, 3.3962) centre (-11.7846, 3.3271) ccw
  line L36 (-11.7957, 3.5809) -> (-10.7394, 3.627)
  arc A61 (-10.7394, 3.627) -> (-10.5159, 3.7836) centre (-10.7505, 3.8808) ccw
  line L37 (-10.5159, 3.7836) -> (-10.1112, 4.7604)
  arc A62 (-10.1112, 4.7604) -> (-10.1586, 5.0292) centre (-10.3459, 4.8576) ccw
  line L38 (-10.1586, 5.0292) -> (-10.8729, 5.8087)
  arc A63 (-10.9073, 6.1044) -> (-10.8729, 5.8087) centre (-10.6856, 5.9803) ccw
  arc A64 (-9.8138, 7.741) -> (-10.9073, 6.1044) centre (0, 0) ccw
  arc A65 (-9.5275, 7.8223) -> (-9.8138, 7.741) centre (-9.6143, 7.5837) ccw
  line L39 (-9.5275, 7.8223) -> (-8.534, 7.4607)
  arc A66 (-8.534, 7.4607) -> (-8.2675, 7.5198) centre (-8.4471, 7.6994) ccw
  line L40 (-8.2675, 7.5198) -> (-7.5198, 8.2675)
  arc A67 (-7.5198, 8.2675) -> (-7.4607, 8.534) centre (-7.6994, 8.4471) ccw
  line L41 (-7.4607, 8.534) -> (-7.8223, 9.5275)
  arc A68 (-7.741, 9.8138) -> (-7.8223, 9.5275) centre (-7.5837, 9.6143) ccw
  arc A69 (-6.1044, 10.9073) -> (-7.741, 9.8138) centre (0, 0) ccw
  arc A70 (-5.8087, 10.8729) -> (-6.1044, 10.9073) centre (-5.9803, 10.6856) ccw
  line L42 (-5.8087, 10.8729) -> (-5.0292, 10.1586)
  arc A71 (-5.0292, 10.1586) -> (-4.7604, 10.1112) centre (-4.8576, 10.3459) ccw
  line L43 (-4.7604, 10.1112) -> (-3.7836, 10.5159)
  arc A72 (-3.7836, 10.5159) -> (-3.627, 10.7394) centre (-3.8808, 10.7505) ccw
  line L44 (-3.627, 10.7394) -> (-3.5809, 11.7957)
  arc A73 (-3.3962, 12.0291) -> (-3.5809, 11.7957) centre (-3.3271, 11.7846) ccw
  arc A74 (-1.4657, 12.4131) -> (-3.3962, 12.0291) centre (0, 0) ccw
  arc A75 (-1.2057, 12.2682) -> (-1.4657, 12.4131) centre (-1.4359, 12.1608) ccw
  line L45 (-1.2057, 12.2682) -> (-0.7589, 11.31)
  arc A76 (-0.7589, 11.31) -> (-0.5287, 11.1633) centre (-0.5287, 11.4173) ccw
  line L46 (-0.5287, 11.1633) -> (0.5287, 11.1633)
  arc A77 (0.5287, 11.1633) -> (0.7589, 11.31) centre (0.5287, 11.4173) ccw
  line L47 (0.7589, 11.31) -> (1.2057, 12.2682)
  arc A78 (1.4657, 12.4131) -> (1.2057, 12.2682) centre (1.4359, 12.1608) ccw
  arc A79 (3.3962, 12.0291) -> (1.4657, 12.4131) centre (0, 0) ccw
  arc A80 (3.5809, 11.7957) -> (3.3962, 12.0291) centre (3.3271, 11.7846) ccw
  circle A81 centre (0, 0) radius 12.5
  dimension "d45" = 25
  dimension "d46" = 0
  dimension "d47" = 0
  dimension "d48" = 0
  dimension "d49" = 0
  constraints: 160 point on circle, 96 end point, 82 centre point, 2 coincident
  measures "d45" diameter of A81
  measures "d46" distance of point (0, 0) A4.centre
  measures "d47" distance of point (0, 0) A4.centre
  measures "d48" distance of point (0, 0) A0.centre
  measures "d49" distance of point (0, 0) A0.centre
extrude "Extrusion5" cut sketch "Sketch6" along normal blind 11.25 contours A80 A81 A3 L2 A2 L1 A1 L0 | A78 L47 A77 L46 A76 L45 A75 A81 | A81 A8 L5 A7 L4 A6 L3 A5 | A73 L44 A72 L43 A71 L42 A70 A81 | A81 A13 L8 A12 L7 A11 L6 A10 | A68 L41 A67 L40 A66 L39 A65 A81 | A81 A18 L11 A17 L10 A16 L9 A15 | A63 L38 A62 L37 A61 L36 A60 A81 | A58 L35 A57 L34 A56 L33 A55 A81 | A81 A23 L14 A22 L13 A21 L12 A20 | A53 L32 A52 L31 A51 L30 A50 A81 | A81 A28 L17 A27 L16 A26 L15 A25 | A48 L29 A47 L28 A46 L27 A45 A81 | A81 A33 L20 A32 L19 A31 L18 A30 | A43 L26 A42 L25 A41 L24 A40 A81 | A81 A38 L23 A37 L22 A36 L21 A35
body "Solid1"
